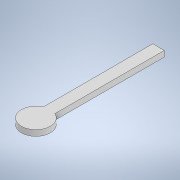
# Autodesk Inventor part: expo13
Saved by Autodesk Inventor 2020 (Build 240168000, 168)
## iProperties
Created: 2020-03-01
Part Number: expo13
Material: Generic
Document SubType Name: Modeling
Designer: Aryan
Density: 1 g/cm^3
Appearance: Default
Author: Aryan
Autodesk Inventor part; units mm, degrees
ref_plane "YZ Plane" through (0, 0, 0) normal (1, 0, 0) x (0, 1, 0)
ref_plane "XZ Plane" through (0, 0, 0) normal (0, 1, 0) x (-1, 0, 0)
ref_plane "XY Plane" through (0, 0, 0) normal (0, 0, 1) x (1, 0, 0)
sketch "Sketch1" plane through (0, 0, 0) normal (0, 1, 0) x (-1, 0, 0)
  point P0 (0, 0)
sketch "Sketch2" plane through (0, 0, 0) normal (0, 1, 0) x (-1, 0, 0)
  point P0 (0, 0)
sketch "Sketch3" plane through (0, 0, 0) normal (0, 1, 0) x (-1, 0, 0)
  circle A0 centre (0, 0) radius 10
  dimension "d0" = 20
  constraints: 1 centre point, 1 coincident
  measures "d0" diameter of A0
extrude "Extrusion1" add sketch "Sketch3" along normal blind 4
sketch "Sketch4" plane through (0, 4, 0) normal (0, 1, 0) x (1, 0, 0)
  line L0 (0, 0) -> (-4, 0)
  line L1 (-4, 0) -> (4, 0)
  line L2 (4, 0) -> (4, 1.5817)
  line L3 (4, 1.5817) -> (-4, 1.5817)
  line L4 (-4, 1.5817) -> (-4, 0)
  line L5 (-4, 0) -> (4, 0)
  line L6 (4, 0) -> (4, 85)
  line L7 (4, 85) -> (-4, 85)
  line L8 (-4, 85) -> (-4, 0)
  dimension "d3" = 4
  dimension "d4" = 8
  dimension "d5" = 8
  dimension "d6" = 85
  constraints: 18 end point, 4 parallel, 3 horizontal, 2 perpendicular
  measures "d3" distance of L0.start L0.end
  measures "d4" distance of L3.end L2.end
  measures "d5" distance of L7.end L6.end
  measures "d6" distance of L6.end L5.end
extrude "Extrusion2" add sketch "Sketch4" against normal blind 4 contours L8 L7 L6 L3
body "Solid1"
